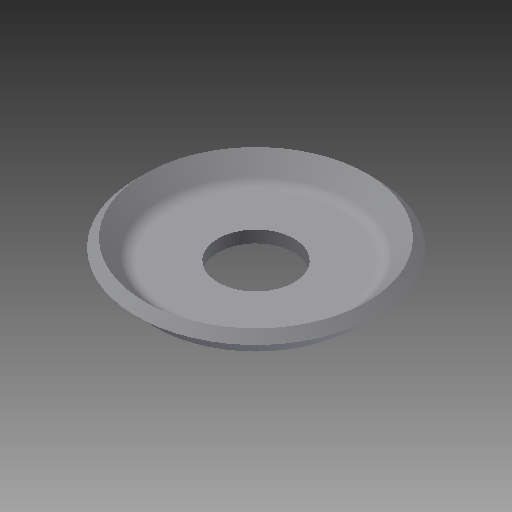
# Autodesk Inventor part: Rondella inferiore
Saved by Autodesk Inventor 2019 (Build 230136000, 136)
## iProperties
Created: 2011-09-21
Part Number: Rondella inferiore
Document SubType Name: Modeling
Designer: Stefano
Density: 1 g/cm^3
Material: 一般
Appearance: 既定
Mass: 1.01121 g
Surface Area: 15.1785 cm^2
Volume: 1.01121 cm^3
Author: Stefano
Autodesk Inventor part; units mm, degrees
ref_plane "YZ Plane" through (0, 0, 0) normal (1, 0, 0) x (0, 1, 0)
ref_plane "XZ Plane" through (0, 0, 0) normal (0, 1, 0) x (-1, 0, 0)
ref_plane "XY Plane" through (0, 0, 0) normal (0, 0, 1) x (1, 0, 0)
sketch "Schizzo1" plane through (0, 0, 0) normal (0, 0, 1) x (1, 0, 0)
  line L0 (4.75, 1.699) -> (10.5858, 1.699)
  line L1 (4.75, 0.199) -> (11.2071, 0.199)
  line L2 (12, 2.2848) -> (13.8891, 4.1739)
  line L3 (12.6213, 0.7848) -> (14.9497, 3.1132)
  line L4 (13.8891, 4.1739) -> (14.9497, 3.1132)
  arc A0 (11.2071, 0.199) -> (12.6213, 0.7848) centre (11.2071, 2.199) ccw
  arc A1 (10.5858, 1.699) -> (12, 2.2848) centre (10.5858, 3.699) ccw
  line L5 (4.75, 1.699) -> (4.75, 0.199)
  line L6 (0, -0.8348) -> (0, 5.0087) projected
  point P0 (0, 0)
  point P1 (11.4142, 1.699)
  dimension "d1" = 1.5
  dimension "d2" = 135
  dimension "d3" = 3.5
  dimension "d4" = 1.5
  dimension "d5" = 2
  constraints: 12 end point, 4 point on circle, 4 tangent, 2 centre point, 2 parallel, 2 perpendicular, 2 point on line, 1 equal radius, 1 horizontal
  measures "d1" distance between parallel lines of L1 L0
  measures "d2" angle of L2 L0
  measures "d3" distance of point (11.414, 1.699) L2.end
  measures "d4" distance between parallel lines of L3 L2
  measures "d5" radius of A0
revolve "Rivoluzione1" add sketch "Schizzo1" angle 360 about axis through (0, -10, 0) along (0, 1, 0)
